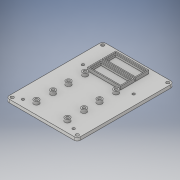
# Autodesk Inventor part: Regulator Mount
Saved by Autodesk Inventor 2019 (Build 230136000, 136)
## iProperties
Created: 2018-11-05
Part Number: Regulator Mount
Material: Generic
Document SubType Name: Modeling
Designer: Keith
Density: 1 g/cm^3
Appearance: Default
Author: Keith
## iProperties of the stored document Regulator Mount_3DPrint.ipt
Created: 2018-11-05
Part Number: Regulator Mount_3DPrint
Material: Generic
Document SubType Name: Modeling
Designer: Keith
Density: 1 g/cm^3
Appearance: Default
Author: Keith
Autodesk Inventor part; units mm, degrees
ref_plane "YZ Plane" through (0, 0, 0) normal (1, 0, 0) x (0, 1, 0)
ref_plane "XZ Plane" through (0, 0, 0) normal (0, 1, 0) x (-1, 0, 0)
ref_plane "XY Plane" through (0, 0, 0) normal (0, 0, 1) x (1, 0, 0)
sketch "Sketch1" plane through (0, 0, 0) normal (0, 1, 0) x (-1, 0, 0)
  line L0 (-3, 3) -> (65.9, 3)
  line L1 (65.9, 3) -> (65.9, -90.5)
  line L2 (65.9, -90.5) -> (-3, -90.5)
  line L3 (-3, -90.5) -> (-3, 3)
  circle A0 centre (62.9, 0) radius 1.55
  circle A1 centre (62.9, -87.5) radius 1.55
  circle A2 centre (0, -87.5) radius 1.55
  circle A3 centre (0, 0) radius 1.55
  constraints: 8 end point, 4 centre point, 2 parallel, 1 coincident, 1 horizontal, 1 perpendicular
extrude "Extrusion1" add sketch "Sketch1" along normal blind 3
sketch "Sketch2" plane through (0, 3, 0) normal (0, 1, 0) x (1, 0, 0)
  circle A0 centre (0, 0) radius 1.55 projected
  circle A1 centre (0, 87.5) radius 1.55 projected
  circle A2 centre (-62.9, 87.5) radius 1.55 projected
  circle A3 centre (-62.9, 0) radius 1.55 projected
  line L0 (-65.9, -3) -> (3, -3) projected
  line L1 (3, -3) -> (3, 90.5) projected
  line L2 (3, 90.5) -> (-65.9, 90.5) projected
  line L3 (-65.9, 90.5) -> (-65.9, -3) projected
  line L4 (3, 90.5) -> (-65.9, 90.5) projected
  circle A4 centre (-46.45, 7) radius 1.35
  circle A5 centre (-46.45, 23) radius 1.35
  circle A6 centre (-16.45, 23) radius 1.35
  circle A7 centre (-16.45, 7) radius 1.35
  circle A8 centre (-16.45, 7) radius 2.5
  circle A9 centre (-16.45, 23) radius 2.5
  circle A10 centre (-46.45, 23) radius 2.5
  circle A11 centre (-46.45, 7) radius 2.5
  constraints: 8 centre point, 8 coincident
extrude "Extrusion2" add sketch "Sketch2" along normal blind 3 contours A8 | A9 | A10 | A11
sketch "Sketch3" plane through (0, 3, 0) normal (0, 1, 0) x (1, 0, 0)
  circle A0 centre (-46.45, 23) radius 2.5 projected
  circle A1 centre (-16.45, 7) radius 2.5 projected
  circle A2 centre (-16.45, 23) radius 2.5 projected
  circle A3 centre (-46.45, 7) radius 2.5 projected
  circle A4 centre (0, 0) radius 1.55 projected
  circle A5 centre (0, 87.5) radius 1.55 projected
  circle A6 centre (-62.9, 87.5) radius 1.55 projected
  circle A7 centre (-62.9, 0) radius 1.55 projected
  line L0 (-65.9, -3) -> (3, -3) projected
  line L1 (3, -3) -> (3, 90.5) projected
  line L2 (3, 90.5) -> (-65.9, 90.5) projected
  line L3 (-65.9, 90.5) -> (-65.9, -3) projected
  circle A8 centre (-46.45, 38) radius 2.5
  circle A9 centre (-46.45, 54) radius 2.5
  circle A10 centre (-16.45, 38) radius 2.5
  circle A11 centre (-16.45, 54) radius 2.5
  circle A12 centre (-46.45, 38) radius 1.35
  circle A13 centre (-46.45, 54) radius 1.35
  circle A14 centre (-16.45, 38) radius 1.35
  circle A15 centre (-16.45, 54) radius 1.35
  dimension "d33" = 5
  dimension "d34" = 5
  dimension "d35" = 5
  dimension "d37" = 15
  dimension "d38" = 15
  dimension "d40" = 16
  dimension "d41" = 2.7
  dimension "d42" = 2.7
  dimension "d44" = 2.7
  dimension "d45" = 2.7
  constraints: 8 centre point, 4 coincident
  measures "d33" diameter of A8
  measures "d34" diameter of A9
  measures "d35" diameter of A10
  measures "d37" distance of A8.centre A0.centre
  measures "d38" distance of A2.centre A10.centre
  measures "d40" distance of A9.centre A8.centre
  measures "d41" diameter of A12
  measures "d42" diameter of A13
  measures "d44" diameter of A14
  measures "d45" diameter of A15
extrude "Extrusion3" add sketch "Sketch3" along normal blind 3 contours A8 | A9 | A10 | A11
sketch "Sketch4" plane through (0, 3, 0) normal (0, 1, 0) x (1, 0, 0)
  circle A0 centre (-16.45, 38) radius 2.5 projected
  circle A1 centre (-46.45, 38) radius 2.5 projected
  circle A2 centre (-46.45, 54) radius 2.5 projected
  circle A3 centre (-16.45, 54) radius 2.5 projected
  circle A4 centre (-46.45, 23) radius 2.5 projected
  circle A5 centre (-16.45, 7) radius 2.5 projected
  circle A6 centre (-16.45, 23) radius 2.5 projected
  circle A7 centre (-46.45, 7) radius 2.5 projected
  circle A8 centre (0, 0) radius 1.55 projected
  circle A9 centre (0, 87.5) radius 1.55 projected
  circle A10 centre (-62.9, 87.5) radius 1.55 projected
  circle A11 centre (-62.9, 0) radius 1.55 projected
  line L0 (-65.9, -3) -> (3, -3) projected
  line L1 (3, -3) -> (3, 90.5) projected
  line L2 (3, 90.5) -> (-65.9, 90.5) projected
  line L3 (-65.9, 90.5) -> (-65.9, -3) projected
  line L4 (-47.6666, 59.5828) -> (-17.6666, 59.5828)
  line L5 (-17.6666, 59.5828) -> (-17.6666, 70.5828)
  line L6 (-17.6666, 70.5828) -> (-47.6666, 70.5828)
  line L7 (-47.6666, 70.5828) -> (-47.6666, 59.5828)
  line L8 (-47.6666, 73.8193) -> (-17.6666, 73.8193)
  line L9 (-17.6666, 73.8193) -> (-17.6666, 84.8193)
  line L10 (-17.6666, 84.8193) -> (-47.6666, 84.8193)
  line L11 (-47.6666, 84.8193) -> (-47.6666, 73.8193)
  line L12 (-48.6666, 58.5828) -> (-16.6666, 58.5828)
  line L13 (-16.6666, 58.5828) -> (-16.6666, 71.5828)
  line L14 (-16.6666, 71.5828) -> (-48.6666, 71.5828)
  line L15 (-48.6666, 71.5828) -> (-48.6666, 58.5828)
  line L16 (-48.6666, 85.8193) -> (-16.6666, 85.8193)
  line L17 (-16.6666, 85.8193) -> (-16.6666, 72.8193)
  line L18 (-16.6666, 72.8193) -> (-48.6666, 72.8193)
  line L19 (-48.6666, 72.8193) -> (-48.6666, 85.8193)
  dimension "d61" = 32
  dimension "d62" = 13
  dimension "d63" = 32
  dimension "d64" = 13
  dimension "d65" = 1
  dimension "d66" = 30
  dimension "d67" = 0
  dimension "d68" = 1
  dimension "d69" = 30
  dimension "d81" = 11
  dimension "d82" = 11
  dimension "d83" = 1
  dimension "d84" = 1
  constraints: 32 end point, 8 parallel, 4 horizontal, 4 perpendicular
  measures "d61" distance of L14.end L13.end
  measures "d62" distance of L13.end L12.end
  measures "d63" distance of L17.end L18.end
  measures "d64" distance of L16.end L17.end
  measures "d65" distance between parallel lines of L19 L11
  measures "d66" distance between parallel lines of L9 L11
  measures "d67" distance between parallel lines of L5 L9
  measures "d68" distance between parallel lines of L7 L15
  measures "d69" distance between parallel lines of L5 L7
  measures "d81" distance of L10.end L8.start
  measures "d82" distance of L6.end L4.start
  measures "d83" distance between parallel lines of L12 L4
  measures "d84" distance between parallel lines of L18 L8
extrude "Extrusion4" add sketch "Sketch4" along normal blind 3 contours L15 L14 L13 L12 | L16 L17 L18 L19
sketch "Sketch5" plane through (0, 3, 0) normal (0, 1, 0) x (1, 0, 0)
  line L0 (-47.6666, 84.8193) -> (-47.6666, 73.8193) projected
  line L1 (-47.6666, 73.8193) -> (-17.6666, 73.8193) projected
  line L2 (-17.6666, 73.8193) -> (-17.6666, 84.8193) projected
  line L3 (-17.6666, 84.8193) -> (-47.6666, 84.8193) projected
  line L4 (-47.6666, 70.5828) -> (-47.6666, 59.5828) projected
  line L5 (-47.6666, 59.5828) -> (-17.6666, 59.5828) projected
  line L6 (-17.6666, 59.5828) -> (-17.6666, 70.5828) projected
  line L7 (-17.6666, 70.5828) -> (-47.6666, 70.5828) projected
  line L8 (-46.6666, 83.8193) -> (-18.6666, 83.8193)
  line L9 (-18.6666, 83.8193) -> (-18.6666, 74.8193)
  line L10 (-18.6666, 74.8193) -> (-46.6666, 74.8193)
  line L11 (-46.6666, 74.8193) -> (-46.6666, 83.8193)
  line L12 (-46.6666, 69.5828) -> (-18.6666, 69.5828)
  line L13 (-18.6666, 69.5828) -> (-18.6666, 60.5828)
  line L14 (-18.6666, 60.5828) -> (-46.6666, 60.5828)
  line L15 (-46.6666, 60.5828) -> (-46.6666, 69.5828)
  point P0 (0, 0)
  dimension "d72" = 1
  dimension "d73" = 1
  dimension "d74" = 1
  dimension "d75" = 1
  dimension "d76" = 1
  dimension "d77" = 1
  constraints: 16 end point, 4 parallel, 2 horizontal, 2 perpendicular, 2 point on line
  measures "d72" distance between parallel lines of L3 L8
  measures "d73" distance between parallel lines of L2 L9
  measures "d74" distance between parallel lines of L1 L10
  measures "d75" distance between parallel lines of L11 L0
  measures "d76" distance between parallel lines of L5 L14
  measures "d77" distance between parallel lines of L7 L12
extrude "Extrusion5" add sketch "Sketch5" along normal blind 2
fillet "Fillet1" radius 3.1 4 edges at (3, 1.5, -90.5) (3, 1.5, 3) (-65.9, 1.5, 3) (-65.9, 1.5, -90.5)
sketch "Sketch6" plane through (0, 3, 0) normal (0, 1, 0) x (1, 0, 0)
  line L0 (-48.6666, 58.5828) -> (-48.6666, 71.5828) projected
  line L1 (-48.6666, 71.5828) -> (-16.6666, 71.5828) projected
  line L2 (-16.6666, 71.5828) -> (-16.6666, 58.5828) projected
  line L3 (-16.6666, 58.5828) -> (-48.6666, 58.5828) projected
  line L4 (-16.6666, 85.8193) -> (-16.6666, 72.8193) projected
  line L5 (-16.6666, 72.8193) -> (-48.6666, 72.8193) projected
  line L6 (-48.6666, 72.8193) -> (-48.6666, 85.8193) projected
  line L7 (-48.6666, 85.8193) -> (-16.6666, 85.8193) projected
  circle A0 centre (-16.45, 38) radius 2.5 projected
  circle A1 centre (-46.45, 38) radius 2.5 projected
  circle A2 centre (-46.45, 54) radius 2.5 projected
  circle A3 centre (-16.45, 54) radius 2.5 projected
  circle A4 centre (-46.45, 23) radius 2.5 projected
  circle A5 centre (-16.45, 7) radius 2.5 projected
  circle A6 centre (-16.45, 23) radius 2.5 projected
  circle A7 centre (-46.45, 7) radius 2.5 projected
  circle A8 centre (0, 0) radius 1.55 projected
  circle A9 centre (0, 87.5) radius 1.55 projected
  circle A10 centre (-62.9, 87.5) radius 1.55 projected
  circle A11 centre (-62.9, 0) radius 1.55 projected
  arc A12 (-62.8, 90.5) -> (-65.9, 87.4) centre (-62.8, 87.4) ccw projected
  line L8 (-65.9, 87.4) -> (-65.9, 0.1) projected
  arc A13 (-65.9, 0.1) -> (-62.8, -3) centre (-62.8, 0.1) ccw projected
  line L9 (-62.8, -3) -> (-0.1, -3) projected
  arc A14 (-0.1, -3) -> (3, 0.1) centre (-0.1, 0.1) ccw projected
  line L10 (3, 0.1) -> (3, 87.4) projected
  arc A15 (3, 87.4) -> (-0.1, 90.5) centre (-0.1, 87.4) ccw projected
  line L11 (-0.1, 90.5) -> (-62.8, 90.5) projected
  circle A16 centre (-55.95, 3.5059) radius 1.25
  circle A17 centre (-6.95, 3.5059) radius 1.25
  circle A18 centre (-6.95, 61.5059) radius 1.25
  circle A19 centre (-55.95, 61.5059) radius 1.25
  dimension "d85" = 2.5
  dimension "d86" = 2.5
  dimension "d87" = 2.5
  dimension "d88" = 2.5
  dimension "d89" = 49
  dimension "d90" = 49
  dimension "d91" = 58
  dimension "d92" = 9.95
  constraints: 4 centre point
  measures "d85" diameter of A16
  measures "d86" diameter of A17
  measures "d87" diameter of A18
  measures "d88" diameter of A19
  measures "d89" distance of A18.centre A19.centre
  measures "d90" distance of A17.centre A16.centre
  measures "d91" distance of A19.centre A16.centre
  measures "d92" distance from line of L8 A16.centre
extrude "Extrusion6" cut sketch "Sketch6" against normal blind 10 contours A16 | A17 | A18 | A19
body "Solid1"
